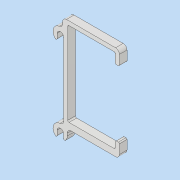
# Autodesk Inventor part: batteryHolderBracket
Saved by Autodesk Inventor 2017 (Build 210142000, 142)
## iProperties
Created: 2019-07-14
Part Number: batteryHolderBracket
Material: ABS Plastic
Document SubType Name: Modeling
Designer: techn
Density: 1.06 g/cm^3
Appearance: Smooth - White
Author: techn
Autodesk Inventor part; units mm, degrees
ref_plane "YZ Plane" through (0, 0, 0) normal (1, 0, 0) x (0, 1, 0)
ref_plane "XZ Plane" through (0, 0, 0) normal (0, 1, 0) x (-1, 0, 0)
ref_plane "XY Plane" through (0, 0, 0) normal (0, 0, 1) x (1, 0, 0)
sketch "Sketch1" plane through (0, 0, 0) normal (0, 0, 1) x (1, 0, 0)
  arc A0 (1.651, 0) -> (-1.651, 0) centre (0, 0) ccw
  arc A1 (1.651, 41.91) -> (-1.651, 41.91) centre (0, 41.91) ccw
  arc A2 (1.143, 45.4111) -> (-1.651, 38.6178) centre (0, 41.91) ccw
  line L0 (3.683, 48.26) -> (27.4676, 48.26)
  line L1 (27.4676, 6.35) -> (3.683, 6.35)
  line L2 (3.683, 6.35) -> (3.683, 48.26)
  line L3 (3.4296, 3.175) -> (3.4296, 0)
  line L4 (1.651, 38.904) -> (1.651, 3.2922)
  line L5 (1.143, 45.4111) -> (1.143, 50.292)
  line L6 (1.143, 50.292) -> (29.4996, 50.292)
  line L7 (29.4996, 50.292) -> (29.4996, 43.18)
  line L8 (29.4996, 43.18) -> (27.4676, 43.18)
  line L9 (3.4296, 3.175) -> (29.4996, 3.175)
  line L10 (29.4996, 3.175) -> (29.4996, 10.16)
  line L11 (29.4996, 10.16) -> (27.4676, 10.16)
  line L12 (27.4676, 48.26) -> (27.4676, 43.18)
  line L13 (27.4676, 10.16) -> (27.4676, 6.35)
  line L14 (1.651, 38.904) -> (1.651, 41.91)
  line L15 (-1.651, 41.91) -> (-1.651, 38.6178)
  line L16 (-1.651, 0) -> (-1.651, -3.2922)
  line L17 (1.651, 0) -> (1.651, -3.006)
  arc A3 (1.651, 3.2922) -> (-1.651, -3.2922) centre (0, 0) ccw
  arc A4 (1.651, -3.006) -> (3.4296, 0) centre (0, 0) ccw
  dimension "d0" = 3.302
  dimension "d2" = 41.91
  dimension "d4" = 6.35
  dimension "d5" = 6.35
  dimension "d6" = 3.683
  dimension "d7" = 2.54
  dimension "d8" = 2.032
  dimension "d9" = 2.032
  dimension "d10" = 5.08
  dimension "d11" = 3.81
  dimension "d12" = 3.175
  dimension "d13" = 2.032
  constraints: 36 end point, 10 point on circle, 9 perpendicular, 6 parallel, 5 centre point, 5 tangent, 4 point on line, 3 coincident, 2 equal radius, 2 horizontal, 1 vertical alignment
  measures "d0" diameter of A0
  measures "d2" distance of point (0, 0) A1.centre
  measures "d4" distance from line of L0 A1.centre
  measures "d5" distance from line of L1 point (0, 0)
  measures "d6" distance from line of A1.centre L2
  measures "d7" distance between parallel lines of L2 L5
  measures "d8" distance between parallel lines of L6 L0
  measures "d9" distance between parallel lines of L12 L7
  measures "d10" distance of L0.end L8.end
  measures "d11" distance of L11.end L1.start
  measures "d12" distance between parallel lines of L1 L9
  measures "d13" distance of L10.end L11.end
extrude "Extrusion1" add sketch "Sketch1" along normal blind 3.81
fillet "Fillet1" radius 0.635 4 edges at (3.683, 48.26, 1.905) (3.683, 6.35, 1.905) (27.4676, 6.35, 1.905) (27.4676, 48.26, 1.905)
fillet "Fillet2" radius 1.905 6 edges at (1.143, 45.4111, 1.905) (1.651, 3.2922, 1.905) (3.4296, 3.175, 1.905) (29.4996, 50.292, 1.905) (1.143, 50.292, 1.905) (29.4996, 3.175, 1.905)
fillet "Fillet3" radius 0.508 3 edges at (1.651, -3.006, 1.905) (-1.651, -3.2922, 1.905) (-1.651, 38.6178, 1.905)
fillet "Fillet4" radius 0.508 4 edges at (27.4676, 10.16, 1.905) (27.4676, 43.18, 1.905) (29.4996, 43.18, 1.905) (29.4996, 10.16, 1.905)
body "Solid1"
